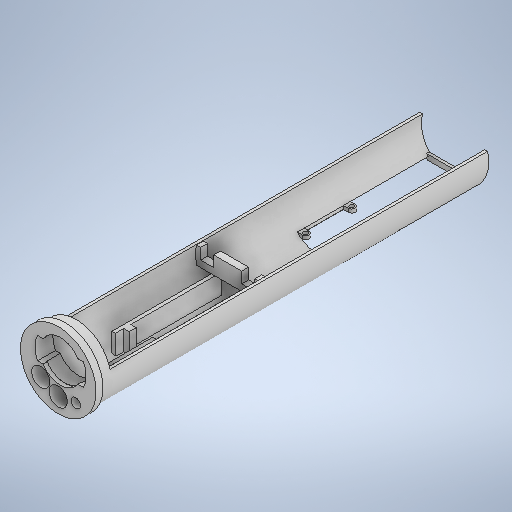
# Autodesk Inventor part: PCB tray CAD
Saved by Autodesk Inventor 2025 (Build 290162000, 162)
## iProperties
Created: 2024-07-01
Part Number: PCB tray CAD
Material: Generic
Document SubType Name: Modeling
Designer: track
Density: 1 g/cm^3
Appearance: Default
Author: track
## iProperties of the stored document PCB tray CAD_3DPrint.ipt
Created: 2024-07-01
Part Number: PCB tray CAD_3DPrint
Material: Generic
Document SubType Name: Modeling
Designer: track
Density: 1 g/cm^3
Appearance: Default
Author: track
Autodesk Inventor part; units mm, degrees
sketch "Sketch9" plane through (0, 0, 0) normal (0, 0, 1) x (1, 0, 0)
  circle A0 centre (0, 0) radius 25.4
  circle A1 centre (0, 0) radius 23.4
  dimension "d29" = 50.8
  dimension "d30" = 2
  constraints: 2 centre point, 2 coincident
  measures "d29" diameter of A0
  measures "d30" radial gap between concentric circles of A0 A1
extrude "Extrusion7" add sketch "Sketch9" against normal blind 287
sketch "Sketch10" plane through (0, 0, 0) normal (0, 0, 1) x (1, 0, 0)
  circle A0 centre (-12.7, -10.541) radius 6.6
  circle A1 centre (0, -16.51) radius 6.65
  circle A2 centre (12.7, -14.224) radius 3.4
  circle A3 centre (0, 0) radius 23.4 projected
  line L0 (18.901, -1.65) -> (-15.599, -1.65) construction
  line L1 (-15.599, -1.65) -> (-15.599, 14.35) construction
  line L2 (-15.599, 14.35) -> (18.901, 14.35) construction
  line L3 (18.901, 14.35) -> (18.901, -1.65) construction
  line L4 (18.901, -1.65) -> (-15.599, 14.35) construction
  line L5 (-15.599, -1.65) -> (18.901, 14.35) construction
  arc A4 (-11.0376, -1.65) -> (14.3396, -1.65) centre (1.651, 6.35) ccw
  arc A5 (14.3396, 14.35) -> (-11.0376, 14.35) centre (1.651, 6.35) ccw
  circle A6 centre (1.651, 6.35) radius 18.5 construction
  arc A7 (18.3318, -1.65) -> (18.3318, 14.35) centre (1.651, 6.35) ccw
  arc A8 (-15.0298, 14.35) -> (-15.0298, -1.65) centre (1.651, 6.35) ccw
  line L6 (-15.0298, 14.35) -> (-11.0376, 14.35)
  line L7 (14.3396, 14.35) -> (18.3318, 14.35)
  line L8 (18.3318, -1.65) -> (14.3396, -1.65)
  line L9 (-11.0376, -1.65) -> (-15.0298, -1.65)
  line L10 (1.651, 6.35) -> (-16.849, 6.35) construction
  line L11 (23.4, 0) -> (-23.4, 0) construction
  line L12 (0, -23.4) -> (0, 23.4) construction
  point P0 (18.901, 13.7954)
  point P1 (17.7647, -15.2307)
  point P2 (0, 0)
  dimension "d33" = 13.2
  dimension "d34" = 13.3
  dimension "d35" = 6.8
  dimension "d90" = 16
  dimension "d91" = 34.5
  dimension "d92" = 15
  dimension "d93" = 15
  dimension "d94" = 37
  dimension "d225" = 0
  dimension "d227" = 0
  dimension "d228" = 6.35
  dimension "d229" = 1.651
  dimension "d230" = 8
  dimension "d231" = 16.51
  dimension "d232" = 12.7
  dimension "d233" = 10.541
  dimension "d234" = 14.224
  dimension "d235" = 12.7
  constraints: 26 end point, 17 point on circle, 9 point on line, 8 centre point, 4 midpoint, 3 collinear, 3 parallel, 2 concentric, 2 horizontal, 1 coincident, 1 perpendicular, 1 vertical
  measures "d33" diameter of A0
  measures "d34" diameter of A1
  measures "d35" diameter of A2
  measures "d90" distance between parallel lines of L2 L0
  measures "d91" distance of L1.end L2.end
  measures "d92" radius of A5
  measures "d93" radius of A4
  measures "d94" diameter of A6
  measures "d225" distance from line of point (0, 0) L11
  measures "d227" distance from line of point (0, 0) L12
  measures "d228" vertical distance of point (0, 0) A4.centre
  measures "d229" horizontal distance of point (0, 0) A4.centre
  measures "d230" distance from line of A6.centre L2
  measures "d231" distance of point (0, 0) A1.centre
  measures "d232" horizontal distance of point (0, 0) A0.centre
  measures "d233" vertical distance of point (0, 0) A0.centre
  measures "d234" vertical distance of point (0, 0) A2.centre
  measures "d235" distance from line of L12 A2.centre
extrude "Extrusion8" add sketch "Sketch10" against normal blind 13
ref_plane "Work Plane1" through (0, 25.4, 0) normal (0, 1, 0) x (-1, 0, 0)
sketch "Sketch11" plane through (0, 25.4, 0) normal (0, 1, 0) x (-1, 0, 0)
  line L0 (-25.4, -287) -> (25.4, -287) projected
  line L1 (-25.4, 0) -> (-25.4, -287) projected
  line L2 (25.4, -287) -> (-25.4, -287)
  line L3 (-25.4, -287) -> (-25.4, -190)
  line L4 (-25.4, -190) -> (25.4, -190)
  line L5 (25.4, -190) -> (25.4, -287)
  point P0 (0, 0)
  dimension "d53" = 97
  constraints: 8 end point, 2 parallel, 1 horizontal, 1 perpendicular, 1 point on line
  measures "d53" distance of L4.end L0.end
extrude "Extrusion9" cut sketch "Sketch11" against normal blind 19.05
sketch "Sketch12" plane through (0, 0, -287) normal (0, 0, -1) x (-1, 0, 0)
  circle A0 centre (0, 0) radius 25.4 projected
  line L0 (-19.2809, -16.535) -> (19.2809, -16.535)
  line L1 (16, -16.535) -> (-16, -16.535) projected
  arc A1 (-19.2809, -16.535) -> (19.2809, -16.535) centre (0, 0) ccw
  dimension "d86" = 16.535
  constraints: 4 point on circle, 2 end point, 1 centre point, 1 concentric, 1 horizontal
  measures "d86" distance from line of A0.centre L0
extrude "Extrusion10" cut sketch "Sketch12" against normal blind 97 contours L0 A0 picked at (1.0399, -19.4259)
ref_plane "Work Plane3" through (0, -16.51, 0) normal (0, 1, 0) x (-1, 0, 0)
sketch "Sketch13" plane through (0, -16.51, 0) normal (0, 1, 0) x (-1, 0, 0)
  line L0 (0, 0) -> (0, -257.1233) construction
  line L1 (-16.5576, -287) -> (-16.5576, -190) projected
  line L2 (-16.5576, -190) -> (-13.0576, -190)
  line L3 (-13.0576, -190) -> (-13.0576, -195) construction
  line L4 (-13.0576, -195) -> (-16.5576, -195)
  line L5 (-16.5576, -195) -> (-16.5576, -190)
  line L6 (16.5576, -190) -> (16.5576, -287) projected
  line L7 (16.5576, -190) -> (13.0576, -190)
  line L8 (13.0576, -190) -> (13.0576, -195) construction
  line L9 (13.0576, -195) -> (16.5576, -195)
  line L10 (16.5576, -195) -> (16.5576, -190)
  line L11 (-16.5576, -223.5) -> (-13.0576, -223.5)
  line L12 (-13.0576, -223.5) -> (-13.0576, -228.5) construction
  line L13 (-13.0576, -228.5) -> (-16.5576, -228.5)
  line L14 (-16.5576, -228.5) -> (-16.5576, -223.5)
  line L15 (16.5576, -223.5) -> (13.0576, -223.5)
  line L16 (13.0576, -223.5) -> (13.0576, -228.5) construction
  line L17 (13.0576, -228.5) -> (16.5576, -228.5)
  line L18 (16.5576, -228.5) -> (16.5576, -223.5)
  arc A0 (-13.0576, -195) -> (-13.0576, -190) centre (-13.0576, -192.5) ccw
  arc A1 (13.0576, -190) -> (13.0576, -195) centre (13.0576, -192.5) ccw
  arc A2 (-13.0576, -228.5) -> (-13.0576, -223.5) centre (-13.0576, -226) ccw
  arc A3 (13.0576, -223.5) -> (13.0576, -228.5) centre (13.0576, -226) ccw
  circle A4 centre (-13.0576, -192.5) radius 1.5
  circle A5 centre (13.0576, -192.5) radius 1.5
  circle A6 centre (-13.0576, -226) radius 1.5
  circle A7 centre (13.0576, -226) radius 1.5
  point P0 (-10.5576, -192.5)
  point P1 (16.5576, -228.5)
  point P2 (16.5576, -223.5)
  point P3 (-16.5576, -223.5)
  point P4 (-16.5576, -228.5)
  dimension "d60" = 5
  dimension "d61" = 5
  dimension "d62" = 28.5
  dimension "d63" = 6
  dimension "d64" = 3
  dimension "d65" = 3
  constraints: 34 end point, 9 point on circle, 8 centre point, 8 parallel, 8 tangent, 5 point on line, 4 coincident, 4 horizontal, 4 perpendicular, 1 vertical, 6 other
  measures "d60" distance of L2.end L3.end
  measures "d61" distance of L11.end L12.end
  measures "d62" distance between parallel lines of L4 L11
  measures "d63" distance from line of L1 point (-10.558, -192.5)
  measures "d64" diameter of A4
  measures "d65" diameter of A6
extrude "Extrusion11" add sketch "Sketch13" against normal blind 2.54
sketch "Sketch14" plane through (0, 0, -190) normal (0, 0, -1) x (-1, 0, 0)
  line L0 (16.5576, -19.05) -> (13.5889, -19.05) projected
  arc A0 (-13.5889, -19.05) -> (13.5889, -19.05) centre (0, 0) ccw projected
  line L1 (-13.5889, -19.05) -> (-16.5576, -19.05) projected
  line L2 (-16.5576, -19.05) -> (-16.5576, -16.535) projected
  line L3 (-19.2809, -16.535) -> (-16.5576, -16.535) projected
  arc A1 (-19.2809, -16.535) -> (19.2809, -16.535) centre (0, 0) ccw projected
  line L4 (16.5576, -16.535) -> (19.2809, -16.535) projected
  line L5 (16.5576, -16.535) -> (16.5576, -19.05) projected
  line L6 (13.0576, -16.51) -> (13.0576, -19.05) projected
  line L7 (13.0576, -19.05) -> (16.8005, -19.05)
  line L8 (-13.0576, -16.51) -> (-13.0576, -19.05) projected
  line L9 (-13.0576, -19.05) -> (-16.8005, -19.05)
  point P0 (-16.5576, -19.2615)
  point P1 (16.5576, -19.2615)
  constraints: 4 end point, 4 point on circle, 3 point on line, 1 perpendicular
extrude "Extrusion12" add sketch "Sketch14" along normal up to surface (38.5 mm away) contours L5 L4 A1 L7 | A1 L3 L2 L9
sketch "Sketch15" plane through (0, 25.4, 0) normal (0, 1, 0) x (-1, 0, 0)
  line L0 (-25.4, 0) -> (-25.4, -287) projected
  line L1 (25.4, 0) -> (25.4, -287) projected
  line L2 (-25.4, -13) -> (25.4, -13)
  line L3 (25.4, -13) -> (25.4, -233)
  line L4 (25.4, -233) -> (-25.4, -233)
  line L5 (-25.4, -233) -> (-25.4, -13)
  line L6 (23.4, -13) -> (-23.4, -13) projected
  point P0 (0, 0)
  point P1 (-25.4, -233)
  point P2 (25.4, -13)
  dimension "d70" = 0
  dimension "d182" = 220
  constraints: 8 end point, 2 parallel, 2 point on line, 1 horizontal, 1 perpendicular
  measures "d70" distance between parallel lines of L6 L2
  measures "d182" distance between parallel lines of L2 L4
extrude "Extrusion13" cut sketch "Sketch15" against normal up to surface (19.05 mm away)
sketch "Sketch17" plane through (0, 0, -287) normal (0, 0, -1) x (-1, 0, 0)
  circle A0 centre (0, 0) radius 25.4
  arc A1 (-16.8005, -19.05) -> (16.8005, -19.05) centre (0, 0) ccw projected
  line L0 (-19.2809, -16.535) -> (-16.5576, -16.535) projected
  line L1 (-20.32, -15.24) -> (20.32, -15.24)
  line L2 (16.5576, -19.05) -> (13.0576, -19.05) projected
  line L3 (-16.8005, -19.05) -> (16.8005, -19.05)
  point P0 (16.8005, -19.05)
  dimension "d74" = 3.81
  constraints: 4 end point, 2 parallel, 2 point on circle, 1 centre point, 1 coincident, 1 concentric
  measures "d74" distance between parallel lines of L1 L3
extrude "Extrusion14" add sketch "Sketch17" against normal blind 2 contours L1 A0 L3 L2
sketch "Sketch18" plane through (0, 0, -13) normal (0, 0, -1) x (-1, 0, 0)
  circle A0 centre (0, 0) radius 27.4
  circle A1 centre (0, 0) radius 25.4
  arc A2 (16.8005, -19.05) -> (24.5934, 6.35) centre (0, 0) ccw projected
  dimension "d87" = 2
  constraints: 2 centre point, 2 coincident, 1 concentric
  measures "d87" radial gap between concentric circles of A0 A1
extrude "Extrusion15" add sketch "Sketch18" along normal blind 5 from surface at -13
sketch "Sketch30" plane through (0, 0, -13) normal (0, 0, -1) x (-1, 0, 0)
  arc A0 (24.5934, 6.35) -> (-24.5934, 6.35) centre (0, 0) ccw projected
  line L0 (9.3, -21.4725) -> (9.3, -6.89)
  line L1 (9.3, -6.89) -> (11.84, -6.89)
  line L2 (11.84, -6.89) -> (11.84, -20.1835)
  line L3 (-6.7, -22.4203) -> (-6.7, -6.89)
  line L4 (-6.7, -6.89) -> (-9.24, -6.89)
  line L5 (-9.24, -6.89) -> (-9.24, -21.4984)
  arc A1 (-13.5889, -19.05) -> (13.5889, -19.05) centre (0, 0) ccw projected
  circle A2 centre (0, 0) radius 23.4
  arc A3 (17.7568, -15.24) -> (22.5219, 6.35) centre (0, 0) ccw projected
  circle A4 centre (0, -16.51) radius 6.65 projected
  point P0 (0, -23.4)
  point P1 (0, -23.4)
  point P2 (12.34, -19.8818)
  point P3 (11.84, -20.1835)
  dimension "d208" = 2.54
  dimension "d247" = 2.54
  dimension "d250" = 16.51
  dimension "d254" = 6.7
  dimension "d308" = 16
  constraints: 12 end point, 5 point on circle, 2 concentric, 2 perpendicular, 2 point on line, 2 vertical, 1 centre point, 1 coincident, 1 parallel
  measures "d208" distance between parallel lines of L2 L0
  measures "d247" distance between parallel lines of L3 L5
  measures "d250" distance from line of point (0, -23.4) L4
  measures "d254" distance from line of A4.centre L3
  measures "d308" distance between parallel lines of L0 L3
extrude "Extrusion23" add sketch "Sketch30" along normal blind 115 contours L0 L1 L2 A1 | A1 L5 L4 L3
sketch "Sketch31" plane through (0, 0, 0) normal (0, 1, 0) x (-1, 0, 0)
  line L0 (-22.5219, -13) -> (-22.5219, -287) projected
  line L1 (22.5219, -287) -> (22.5219, -13) projected
  line L2 (-22.5219, -13) -> (22.5219, -13)
  line L3 (22.5219, -13) -> (22.5219, -23)
  line L4 (22.5219, -23) -> (-22.5219, -23)
  line L5 (-22.5219, -23) -> (-22.5219, -13)
  point P0 (0, 0)
  dimension "d183" = 10
  constraints: 8 end point, 2 parallel, 1 horizontal, 1 perpendicular, 1 point on line
  measures "d183" distance between parallel lines of L2 L4
extrude "Extrusion24" cut sketch "Sketch31" against normal up to surface round surface about axis through (0, 0, 0) along (0, 0, -1) radius 23.4 far side no
sketch "Sketch36" plane through (0, 0, -128) normal (0, 0, -1) x (-1, 0, 0)
  arc A0 (-22.5219, 6.35) -> (-17.7568, -15.24) centre (0, 0) ccw projected
  line L0 (-22.3626, -6.89) -> (22.3626, -6.89)
  arc A1 (17.7568, -15.24) -> (22.5219, 6.35) centre (0, 0) ccw projected
  line L1 (-22.6672, 5.81) -> (22.6672, 5.81)
  line L2 (4.7625, -6.89) -> (3.4925, -6.89)
  line L3 (11.84, -6.89) -> (9.3, -6.89) projected
  dimension "d212" = 12.7
  constraints: 6 end point, 4 point on circle, 2 collinear, 2 horizontal
  measures "d212" distance between parallel lines of L1 L0
extrude "Extrusion28" add sketch "Sketch36" against normal blind 5
sketch "Sketch37" plane through (0, 0, -128) normal (0, 0, -1) x (-1, 0, 0)
  line L0 (-22.6672, 5.81) -> (22.6672, 5.81) projected
  line L1 (-19.8754, 5.81) -> (-9.8754, 5.81)
  line L2 (10.1246, 5.81) -> (20.1246, 5.81)
  line L3 (-19.66, 5.81) -> (-10.16, 5.81)
  line L4 (-10.16, 5.81) -> (-10.16, -2.19)
  line L5 (-10.16, -2.19) -> (-19.66, -2.19)
  line L6 (-19.66, -2.19) -> (-19.66, 5.81)
  line L7 (10.16, 5.81) -> (19.66, 5.81)
  line L8 (19.66, 5.81) -> (19.66, -2.19)
  line L9 (19.66, -2.19) -> (10.16, -2.19)
  line L10 (10.16, -2.19) -> (10.16, 5.81)
  point P0 (0, 0)
  dimension "d258" = 9.5
  dimension "d259" = 8
  dimension "d260" = 10.16
  dimension "d261" = 8
  dimension "d262" = 9.5
  dimension "d263" = 10.16
  constraints: 20 end point, 6 point on line, 4 parallel, 2 collinear, 2 horizontal, 2 perpendicular
  measures "d258" distance between parallel lines of L6 L4
  measures "d259" distance of L3.end L4.end
  measures "d260" distance from line of point (0, 0) L4
  measures "d261" distance of L9.end L7.start
  measures "d262" distance between parallel lines of L8 L10
  measures "d263" distance from line of point (0, 0) L10
extrude "Extrusion29" cut sketch "Sketch37" against normal up to surface (5 mm away)
sketch "Sketch44" plane through (0, 0, 0) normal (0, 0, 1) x (1, 0, 0)
  line L0 (-15.0298, 14.35) -> (-11.0376, 14.35) projected
  arc A0 (14.3396, 14.35) -> (-11.0376, 14.35) centre (1.651, 6.35) ccw projected
  line L1 (14.3396, 14.35) -> (18.3318, 14.35) projected
  arc A1 (18.3318, -1.65) -> (18.3318, 14.35) centre (1.651, 6.35) ccw projected
  line L2 (18.3318, -1.65) -> (14.3396, -1.65) projected
  arc A2 (-11.0376, -1.65) -> (14.3396, -1.65) centre (1.651, 6.35) ccw projected
  line L3 (-11.0376, -1.65) -> (-15.0298, -1.65) projected
  arc A3 (-15.0298, 14.35) -> (-15.0298, -1.65) centre (1.651, 6.35) ccw projected
  circle A4 centre (12.7, -14.224) radius 3.4 projected
  circle A5 centre (0, -16.51) radius 6.65 projected
  circle A6 centre (-12.7, -10.541) radius 6.6 projected
  circle A7 centre (0, 0) radius 27.4 projected
extrude "Extrusion33" cut sketch "Sketch44" against normal blind 28 contours A4 | A6
sketch "Sketch46" plane through (-9.3, -6.89, -28) normal (0, 1, 0) x (1, 0, 0)
  line L0 (0, 0) -> (-2.54, 0) projected
  line L1 (0, -5) -> (-2.54, -5) projected
  line L2 (-2.54, 0) -> (0, 0)
  line L3 (0, 0) -> (0, -5)
  line L4 (0, -5) -> (-2.54, -5)
  line L5 (-2.54, -5) -> (-2.54, 0)
  point P0 (9.3, -28)
  constraints: 8 end point, 2 parallel, 1 horizontal, 1 perpendicular
extrude "Extrusion34" cut sketch "Sketch46" against normal up to surface round surface about axis through (0, 0, 0) along (0, 0, -1) radius 23.4 far side no
ref_plane "Work Plane5" through (13.0175, -7.4, -25) normal (0, 1, 0) x (1, 0, 0)
sketch "Sketch49" plane through (6.7, -6.89, -23) normal (0, 1, 0) x (1, 0, 0)
  line L0 (-16, 5) -> (-16, 100) projected
  line L1 (-16, 38.9) -> (-12, 38.9)
  line L2 (-12, 38.9) -> (-12, 33.9)
  line L3 (-12, 33.9) -> (-16, 33.9)
  line L4 (-16, 33.9) -> (-16, 38.9)
  line L5 (6.8889, 167) -> (-20.2889, 167) projected
  line L6 (0, 0) -> (0, 100) projected
  line L7 (20.7, -23) -> (-34.1, -23) projected
  point P0 (-6.7, -23)
  point P1 (-16, 33.9)
  dimension "d266" = 12
  dimension "d267" = 61.9
  dimension "d268" = 5
  constraints: 8 end point, 2 parallel, 1 horizontal, 1 perpendicular, 1 point on line
  measures "d266" distance between parallel lines of L6 L2
  measures "d267" distance between parallel lines of L7 L1
  measures "d268" distance between parallel lines of L1 L3
extrude "Extrusion36" add sketch "Sketch49" against normal up to surface round surface about axis through (0, 0, 0) along (0, 0, -1) radius 23.4 far side no
ref_plane "Work Plane6" through (-11.84, 3.11, -123) normal (0, 1, 0) x (1, 0, 0)
sketch "Sketch54" plane through (-11.84, -6.89, -123) normal (0, 1, 0) x (1, 0, 0)
  line L0 (0, -95) -> (0, 0) projected
  line L1 (2.54, -95) -> (2.54, -66.1) projected
  line L2 (0, -95) -> (2.54, -95)
  line L3 (2.54, -95) -> (2.54, -85)
  line L4 (2.54, -85) -> (0, -85)
  line L5 (0, -85) -> (0, -95)
  point P0 (11.84, -123)
  point P1 (2.54, -95)
  point P2 (0, -85)
  dimension "d288" = 10
  constraints: 8 end point, 2 parallel, 1 horizontal, 1 perpendicular, 1 point on line
  measures "d288" distance between parallel lines of L2 L4
extrude "Extrusion40" cut sketch "Sketch54" against normal up to surface round surface about axis through (0, 0, 0) along (0, 0, -1) radius 23.4 far side no
sketch "Sketch55" plane through (0, 0, -128) normal (0, 0, -1) x (-1, 0, 0)
  arc A0 (-22.6672, 5.81) -> (-22.3626, -6.89) centre (0, 0) ccw projected
  line L0 (-9.24, -6.89) -> (-6.7, -6.89) projected
  line L1 (-9.24, -6.89) -> (-6.7, -6.89)
  arc A1 (-22.5219, 6.35) -> (-17.7568, -15.24) centre (0, 0) ccw projected
  arc A2 (-13.5889, -19.05) -> (13.5889, -19.05) centre (0, 0) ccw projected
  line L2 (10.16, -2.19) -> (10.16, 5.81) projected
  line L3 (10.16, 5.81) -> (-10.16, 5.81) projected
  line L4 (-10.16, 5.81) -> (-10.16, -2.19) projected
  line L5 (-10.16, -2.19) -> (-19.66, -2.19) projected
  line L6 (-19.66, -2.19) -> (-19.66, 5.81) projected
  line L7 (-19.66, 5.81) -> (-22.6672, 5.81) projected
  line L8 (-22.3626, -6.89) -> (-9.24, -6.89) projected
  line L9 (-9.24, -6.89) -> (-9.24, -21.4984) projected
  arc A3 (-9.24, -21.4984) -> (-6.7, -22.4203) centre (0, 0) ccw projected
  line L10 (-6.7, -22.4203) -> (-6.7, -6.89) projected
  line L11 (11.84, -6.89) -> (22.3626, -6.89) projected
  arc A4 (22.3626, -6.89) -> (22.6672, 5.81) centre (0, 0) ccw projected
  line L12 (22.6672, 5.81) -> (19.66, 5.81) projected
  line L13 (19.66, 5.81) -> (19.66, -2.19) projected
  line L14 (19.66, -2.19) -> (10.16, -2.19) projected
  line L15 (-6.7, -6.89) -> (9.3, -6.89) projected
  line L16 (9.3, -6.89) -> (9.3, -21.4725) projected
  arc A5 (9.3, -21.4725) -> (11.84, -20.1835) centre (0, 0) ccw projected
  line L17 (11.84, -20.1835) -> (11.84, -6.89) projected
  point P0 (-22.7919, 5.3)
  point P1 (-22.1991, -7.4)
  point P2 (11.7475, -20.2375)
  point P3 (-6.7, -22.4203)
  point P4 (-6.7, -6.89)
  constraints: 2 end point, 1 collinear
extrude "Extrusion41" cut sketch "Sketch55" against normal up to surface (66.1 mm away) contours L0 L10 A2 L9
ref_plane "Work Plane7" through (6.7, -7.4, -28) normal (0, 1, 0) x (1, 0, 0)
sketch "Sketch56" plane through (6.7, -7.4, -28) normal (0, 1, 0) x (1, 0, 0)
  line L0 (5.04, 31.36) -> (0, 31.36)
  line L1 (5.04, 100) -> (2.5, 100)
  line L2 (0, -5) -> (0, 33.9) projected
  line L3 (0, 31.36) -> (0, 33.9)
  line L4 (0, 33.9) -> (2.5, 33.9)
  line L5 (-16, 95) -> (15.6626, 95) projected
  line L6 (5.04, 100) -> (5.04, 31.36)
  line L7 (2.5, 33.9) -> (2.5, 100)
  line L8 (-16.86, 100) -> (3.46, 100) projected
  point P0 (-6.7, -28)
  dimension "d314" = 2.5
  dimension "d315" = 2.54
  dimension "d317" = 2.54
  dimension "d318" = 0
  constraints: 12 end point, 3 perpendicular, 1 collinear
  measures "d314" distance of L2.end L4.end
  measures "d315" distance between parallel lines of L4 L0
  measures "d317" distance between parallel lines of L7 L6
  measures "d318" distance between parallel lines of L8 L1
extrude "Extrusion42" add sketch "Sketch56" against normal up to surface from surface at 0.51 round surface about axis through (0, 0, 0) along (0, 0, -1) radius 23.4 far side no
ref_plane "Work Plane8" through (23.2551, 2.6, -28) normal (0, 0, -1) x (-1, 0, 0)
sketch "Sketch59" plane through (-11.84, -6.89, -123) normal (0, 1, 0) x (1, 0, 0)
  line L0 (2.54, -85) -> (2.54, -66.1) projected
  line L1 (0, -85) -> (0, 0) projected
  line L2 (2.54, -85) -> (0, -85)
  line L3 (0, -85) -> (0, -72.3)
  line L4 (0, -72.3) -> (2.54, -72.3)
  line L5 (2.54, -72.3) -> (2.54, -85)
  line L6 (0, -85) -> (2.54, -85) projected
  point P0 (11.84, -123)
  point P1 (2.54, -72.3)
  dimension "d309" = 12.7
  dimension "d310" = 0
  constraints: 8 end point, 2 parallel, 2 point on line, 1 horizontal, 1 perpendicular
  measures "d309" distance between parallel lines of L4 L2
  measures "d310" distance between parallel lines of L6 L2
extrude "Extrusion45" cut sketch "Sketch59" against normal up to surface round surface about axis through (0, 0, 0) along (0, 0, -1) radius 23.4 far side no
sketch "Sketch60" plane through (0, 0, -13) normal (0, 0, -1) x (-1, 0, 0)
  arc A0 (11.0376, 14.35) -> (-14.3396, 14.35) centre (-1.651, 6.35) ccw projected
  arc A1 (-14.3396, -1.65) -> (11.0376, -1.65) centre (-1.651, 6.35) ccw projected
  circle A2 centre (-1.651, 6.35) radius 15
  circle A3 centre (-1.651, 6.35) radius 15.367
  point P0 (0, 0)
  point P1 (-14.3396, -1.65)
  point P2 (-14.3396, 14.35)
  point P3 (11.0376, -1.65)
  dimension "d319" = 30.734
  dimension "d320" = 15
  constraints: 2 centre point, 1 coincident, 1 concentric
  measures "d319" diameter of A3
  measures "d320" radius of A0
extrude "Extrusion46" cut sketch "Sketch60" against normal blind 10
body "Solid2"
